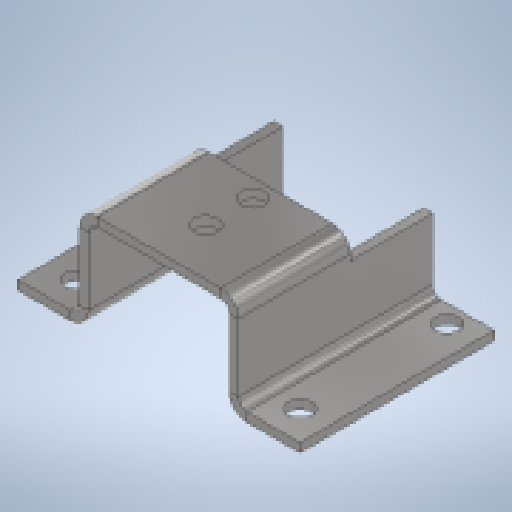
# Autodesk Inventor part: Giá đỡ
Saved by Autodesk Inventor 2023 (Build 270158000, 158)
## iProperties
Created: 2023-10-04
Part Number: Giá đỡ
Material: Steel, Carbon
Document SubType Name: Sheet Metal
Designer: huy20
Density: 7.85 g/cm^3
Sheet Metal Rule: Default_mm
Appearance: Semi-Polished
Author: huy20
Autodesk Inventor part; units mm, degrees
ref_plane "YZ Plane" through (0, 0, 0) normal (1, 0, 0) x (0, 1, 0)
ref_plane "XZ Plane" through (0, 0, 0) normal (0, 1, 0) x (-1, 0, 0)
ref_plane "XY Plane" through (0, 0, 0) normal (0, 0, 1) x (1, 0, 0)
sketch "Sketch1" plane through (0, 0, 0) normal (0, 0, 1) x (1, 0, 0)
  line L0 (-11.9627, 0) -> (-11.9627, 16.0422)
  line L1 (-11.9627, 16.0422) -> (12.0373, 16.0422)
  line L2 (12.0373, 16.0422) -> (12.0373, 0.0422)
  line L3 (12.0373, 0.0422) -> (24.0373, 0.0422)
  line L4 (-11.9627, 0) -> (-23.9627, 0)
  point P0 (0, 0)
  dimension "d0" = 24
  dimension "d1" = 16
  dimension "d2" = 12
  dimension "d3" = 12
  measures "d0" distance between parallel lines of L2 L0
  measures "d1" distance of L1.end L2.end
  measures "d2" distance of L2.end L3.end
  measures "d3" distance of L0.start L4.end
contour flange "Contour Flange1" sketch "Sketch1" thickness 1.5 bend radius 1.5 width 33 along (0, 0, 1) mid plane no both sides no wall seen from (18.0373, 0.0422, 0) lies toward (0, 1, 0) curves L3 L2 L1 L0 L4
bend "Bend1"
corner "Corner1"
sketch "Sketch2" plane through (-10.4627, 17.5422, 33) normal (0, 1, 0) x (1, 0, 0)
  line L0 (-3, 0) -> (-3, 33) projected
  line L1 (24.1789, 19) -> (-3, 19)
  line L2 (-3, 19) -> (-3, 33)
  line L3 (-3, 33) -> (24.1789, 33)
  line L4 (24.1789, 33) -> (24.1789, 19)
  point P0 (10.4627, 33)
  point P1 (10.5895, 33)
  point P2 (10.5895, 19)
  dimension "d15" = 14
  constraints: 8 end point, 2 midpoint, 2 parallel, 1 horizontal, 1 perpendicular
  measures "d15" distance of point (10.589, 33) point (10.589, 19)
extrude "Cut1" cut sketch "Sketch2" against normal blind 4
sketch "Sketch3" plane through (0, 0, 0) normal (0, 1, 0) x (-1, 0, 0)
  line L0 (-15.0373, 33) -> (-15.0373, 0) construction
  line L1 (-24.0373, 33) -> (-15.0373, 33) construction
  line L2 (-24.0373, 0) -> (-24.0373, 33) construction
  line L3 (-24.0373, 0) -> (-15.0373, 0) construction
  line L4 (-10.5373, 14) -> (10.4627, 14) construction
  line L5 (10.4627, 33) -> (10.4627, 14) construction
  line L6 (-10.5373, 33) -> (10.4627, 33) construction
  line L7 (-10.5373, 33) -> (-10.5373, 14) construction
  line L8 (14.9627, 33) -> (14.9627, 0) construction
  line L9 (14.9627, 0) -> (23.9627, 0) construction
  line L10 (23.9627, 0) -> (23.9627, 33) construction
  line L11 (14.9627, 33) -> (23.9627, 33) construction
  point P0 (0, 0)
  point P1 (-0.0373, 25)
  point P2 (-0.0373, 17)
  point P3 (-19.0373, 28)
  point P4 (-19.0373, 3)
  point P5 (18.9627, 28)
  point P6 (18.9627, 3)
  point P7 (-0.0373, 33)
  dimension "d18" = 8
  dimension "d19" = 8
  dimension "d20" = 5
  dimension "d21" = 5
  dimension "d22" = 5
  dimension "d23" = 25
  dimension "d24" = 25
  dimension "d25" = 5
  dimension "d26" = 24
  dimension "d27" = 24
  constraints: 2 horizontal alignment, 2 vertical alignment, 1 midpoint
  measures "d18" distance of point (-0.037, 25) point (-0.037, 17)
  measures "d19" distance of point (-0.037, 33) point (-0.037, 25)
  measures "d20" distance from line of L10 point (18.963, 28)
  measures "d21" distance from line of L2 point (-19.037, 28)
  measures "d22" distance from line of L11 point (18.963, 28)
  measures "d23" distance of point (18.963, 28) point (18.963, 3)
  measures "d24" distance of point (-19.037, 3) point (-19.037, 28)
  measures "d25" distance from line of L1 point (-19.037, 28)
  measures "d26" distance from line of point (-0.037, 25) L10
  measures "d27" distance from line of point (-0.037, 17) L10
hole "Hole1" at (0.0373, 0, 25) at (0.0373, 0, 17) at (-18.9627, 0, 28) at (-18.9627, 0, 3) at (19.0373, 0, 28) at (19.0373, 0, 3) direction (0, 1, 0) diameter 4 end through all
equation "\"d33\" = Thickness"
equation "\"d4\" = Thickness"
equation "\"d5\" = BendReliefWidth"
equation "\"d6\" = BendReliefDepth"
equation "\"d7\" = MinimumRemnant"
equation "\"d8\" = TransitionRadius"
equation "\"d10\" = BendRadius"
equation "\"d12\" = CornerReliefSize"
equation "\"d13\" = GapSize"
equation "\"d14\" = JacobiRadiusSize"
equation "\"BendRadius\" = Thickness"
equation "\"BendReliefWidth\" = Thickness"
equation "\"BendReliefDepth\" = 0.5 * Thickness"
equation "\"CornerReliefSize\" = 4 * Thickness"
equation "\"MinimumRemnant\" = 2 * Thickness"
equation "\"TransitionRadius\" = BendRadius"
equation "\"JacobiRadiusSize\" = BendRadius"
equation "\"GapSize\" = Thickness"
equation "\"Thickness\" = 1.5"
body "Solid1"
